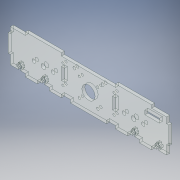
# Autodesk Inventor part: Soporte_Motor
Saved by Autodesk Inventor 2019 (Build 230136000, 136)
## iProperties
Created: 2020-04-02
Part Number: Soporte_Motor
Material: Generic
Document SubType Name: Modeling
Designer: Jurgen
Density: 1 g/cm^3
Appearance: Clear
Author: Jurgen
Autodesk Inventor part; units mm, degrees
ref_plane "YZ Plane" through (0, 0, 0) normal (1, 0, 0) x (0, 1, 0)
ref_plane "XZ Plane" through (0, 0, 0) normal (0, 1, 0) x (-1, 0, 0)
ref_plane "XY Plane" through (0, 0, 0) normal (0, 0, 1) x (1, 0, 0)
sketch "Sketch1" plane through (0, 0, 0) normal (0, 0, 1) x (1, 0, 0)
  arc A0 (19, -20) -> (20, -19) centre (19, -19) ccw construction
  line L0 (20, -19) -> (20, 19) construction
  arc A1 (20, 19) -> (19, 20) centre (19, 19) ccw construction
  line L1 (19, 20) -> (-19, 20) construction
  arc A2 (-19, 20) -> (-20, 19) centre (-19, 19) ccw construction
  line L2 (-20, 19) -> (-20, -19) construction
  arc A3 (-20, -19) -> (-19, -20) centre (-19, -19) ccw construction
  line L3 (-19, -20) -> (19, -20) construction
  circle A4 centre (-15.5, -15.5) radius 2
  circle A5 centre (15.5, -15.5) radius 2.2846
  circle A6 centre (15.5, 15.5) radius 2
  circle A7 centre (-15.5, 15.5) radius 2
  circle A8 centre (0, 0) radius 11
  line L4 (150, -20) -> (150, 20)
  line L5 (150, 20) -> (-150, 20)
  line L6 (-150, 20) -> (-150, -20)
  line L7 (-150, -20) -> (150, 20) construction
  line L8 (150, -20) -> (-150, 20) construction
  line L9 (50, -20) -> (100, -20) construction
  line L10 (100, -20) -> (100, -25)
  line L11 (100, -25) -> (50, -25)
  line L12 (50, -25) -> (50, -20)
  line L13 (100, -20) -> (150, -20)
  line L14 (-150, -20) -> (50, -20) construction
  line L15 (-150, -20) -> (-100, -20)
  line L16 (-100, -20) -> (-100, -25)
  line L17 (-100, -25) -> (-50, -25)
  line L18 (-50, -25) -> (-50, -20)
  line L19 (-50, -20) -> (50, -20)
  circle A9 centre (-91, 0) radius 3
  circle A10 centre (-59, 0) radius 3
  circle A11 centre (59, 0) radius 3
  circle A12 centre (91, 0) radius 3
  circle A13 centre (-75, 0) radius 4
  circle A14 centre (75, 0) radius 4
  dimension "d0" = 300
  dimension "d3" = 50
  dimension "d4" = 5
  dimension "d6" = 50
  dimension "d8" = 50
  dimension "d9" = 50
  dimension "d12" = 6
  dimension "d13" = 6
  dimension "d14" = 32
  dimension "d15" = 6
  dimension "d16" = 6
  dimension "d17" = 32
  dimension "d18" = 59
  dimension "d19" = 59
  dimension "d22" = 8
  dimension "d23" = 8
  dimension "d24" = 16
  dimension "d25" = 16
  constraints: 40 end point, 15 centre point, 8 point on circle, 5 perpendicular, 3 midpoint, 3 parallel, 2 horizontal, 2 point on line, 1 collinear
  measures "d0" distance of L5.end L4.end
  measures "d3" distance of L10.end L11.end
  measures "d4" distance of L9.end L10.end
  measures "d6" distance between parallel lines of L4 L10
  measures "d8" distance of L6.end L15.end
  measures "d9" distance of L16.end L17.end
  measures "d12" diameter of A9
  measures "d13" diameter of A10
  measures "d14" distance of A10.centre A9.centre
  measures "d15" diameter of A11
  measures "d16" diameter of A12
  measures "d17" distance of A12.centre A11.centre
  measures "d18" distance of point (0, 0) A10.centre
  measures "d19" distance of point (0, 0) A11.centre
  measures "d22" diameter of A13
  measures "d23" diameter of A14
  measures "d24" distance of A10.centre A13.centre
  measures "d25" distance of A14.centre A11.centre
extrude "Extrusion3" add sketch "Sketch1" along normal blind 5
sketch "Sketch2" plane through (0, 0, 5) normal (0, 0, 1) x (1, 0, 0)
  circle A0 centre (0, 0) radius 11 construction
  circle A1 centre (75, 0) radius 4 construction
  circle A2 centre (-75, 0) radius 4 construction
  circle A3 centre (91, 0) radius 3 construction
  circle A4 centre (59, 0) radius 3 construction
  circle A5 centre (-59, 0) radius 3 construction
  circle A6 centre (-91, 0) radius 3 construction
  circle A7 centre (15.5, -15.5) radius 2.2846 construction
  circle A8 centre (-15.5, 15.5) radius 2 construction
  circle A9 centre (15.5, 15.5) radius 2 construction
  circle A10 centre (-15.5, -15.5) radius 2 construction
  line L0 (-150, 20) -> (-150, -20) construction
  line L1 (-150, -20) -> (-100, -20) construction
  line L2 (-100, -20) -> (-100, -25) construction
  line L3 (-100, -25) -> (-50, -25) construction
  line L4 (-50, -25) -> (-50, -20) construction
  line L5 (-50, -20) -> (50, -20) construction
  line L6 (50, -20) -> (50, -25) construction
  line L7 (50, -25) -> (100, -25) construction
  line L8 (100, -25) -> (100, -20) construction
  line L9 (100, -20) -> (150, -20) construction
  line L10 (150, -20) -> (150, 20) construction
  line L11 (150, 20) -> (-150, 20) construction
  line L12 (150, 20) -> (-150, 20) construction
  line L13 (-150, 20) -> (150, 20)
  line L14 (150, 20) -> (150, 30)
  line L15 (-150, 30) -> (-150, 20)
  line L16 (-45, 30) -> (-45, 35)
  line L17 (-45, 35) -> (-105, 35) construction
  line L18 (-105, 35) -> (-105, 30)
  line L19 (45, 30) -> (45, 35)
  line L20 (45, 35) -> (105, 35) construction
  line L21 (105, 35) -> (105, 30)
  line L22 (-105, 30) -> (-150, 30)
  line L23 (150, 30) -> (105, 30)
  line L24 (45, 30) -> (-45, 30)
  line L25 (-105, 35) -> (-85, 35)
  line L26 (-65, 35) -> (-45, 35)
  line L27 (45, 35) -> (65, 35)
  line L28 (85, 35) -> (105, 35)
  line L29 (-85, 35) -> (-65, 35)
  line L30 (65, 35) -> (85, 35)
  point P0 (-120, 20)
  point P1 (70, 20)
  dimension "d42" = 10
  dimension "d43" = 5
  dimension "d44" = 5
  dimension "d57" = 45
  dimension "d58" = 90
  dimension "d59" = 45
  constraints: 36 end point, 6 parallel, 6 point on line, 2 collinear, 2 horizontal, 1 perpendicular
  measures "d42" distance of L14.end L13.end
  measures "d43" distance of L16.end L16.start
  measures "d44" distance of L19.start L19.end
  measures "d57" distance between parallel lines of L21 L14
  measures "d58" distance between parallel lines of L16 L19
  measures "d59" distance between parallel lines of L15 L18
extrude "Extrusion6" add sketch "Sketch2" against normal blind 5
sketch "Sketch4" plane through (0, 0, 5) normal (0, 0, 1) x (1, 0, 0)
  circle A0 centre (0, 0) radius 11 construction
  circle A1 centre (75, 0) radius 4 construction
  circle A2 centre (-75, 0) radius 4 construction
  circle A3 centre (91, 0) radius 3 construction
  circle A4 centre (59, 0) radius 3 construction
  circle A5 centre (-59, 0) radius 3 construction
  circle A6 centre (-91, 0) radius 3 construction
  circle A7 centre (15.5, -15.5) radius 2.2846 construction
  circle A8 centre (-15.5, 15.5) radius 2 construction
  circle A9 centre (15.5, 15.5) radius 2 construction
  circle A10 centre (-15.5, -15.5) radius 2 construction
  line L0 (-150, 30) -> (-150, -20) construction
  line L1 (-150, -20) -> (-100, -20) construction
  line L2 (-100, -20) -> (-100, -25) construction
  line L3 (-100, -25) -> (-50, -25) construction
  line L4 (-50, -25) -> (-50, -20) construction
  line L5 (-50, -20) -> (50, -20) construction
  line L6 (50, -20) -> (50, -25) construction
  line L7 (50, -25) -> (100, -25) construction
  line L8 (100, -25) -> (100, -20) construction
  line L9 (100, -20) -> (150, -20) construction
  line L10 (150, -20) -> (150, 30) construction
  line L11 (150, 30) -> (105, 30) construction
  line L12 (105, 30) -> (105, 35) construction
  line L13 (45, 35) -> (45, 30) construction
  line L14 (45, 30) -> (-45, 30) construction
  line L15 (-45, 30) -> (-45, 35) construction
  line L16 (-105, 35) -> (-105, 30) construction
  line L17 (-105, 30) -> (-150, 30) construction
  line L18 (-45, 0) -> (-45, 15) construction
  line L19 (-45, 15) -> (-40, 15) construction
  line L20 (-40, 15) -> (-40, -5) construction
  line L21 (-40, 15) -> (-45, 15)
  line L22 (-45, 15) -> (-45, -5)
  line L23 (-45, -5) -> (-40, -5)
  line L24 (-40, -5) -> (-40, 15)
  line L25 (45, 30) -> (-45, 30) construction
  line L26 (0, 30) -> (0, -20) construction
  line L27 (-50, -20) -> (50, -20) construction
  line L28 (45, 0) -> (45, 15) construction
  line L29 (45, 15) -> (40, 15) construction
  line L30 (40, 15) -> (40, -5) construction
  line L31 (40, 15) -> (45, 15)
  line L32 (45, 15) -> (45, -5)
  line L33 (45, -5) -> (40, -5)
  line L34 (40, -5) -> (40, 15)
  line L35 (105, 35) -> (45, 35) projected
  line L36 (-45, 35) -> (-105, 35) projected
  line L37 (0, 0) -> (-150, 0) construction
  line L38 (-150, 30) -> (-150, -20) construction
  line L39 (-42.5, 15) -> (-42.5, -5) construction
  line L40 (-42.5, 15) -> (-42.5, 30) construction
  line L41 (-45, 30) -> (45, 30) construction
  line L42 (-42.5, -5) -> (-42.5, -20) construction
  circle A11 centre (-42.5, -11) radius 2
  circle A12 centre (-42.5, 21) radius 2
  line L43 (45, 0) -> (45, 15) construction
  line L44 (45, 15) -> (40, 15) construction
  line L45 (40, 15) -> (40, -5) construction
  line L46 (40, 15) -> (45, 15)
  line L47 (45, 15) -> (45, -5)
  line L48 (45, -5) -> (40, -5)
  line L49 (40, -5) -> (40, 15)
  line L50 (42.5, 15) -> (42.5, -5) construction
  circle A13 centre (42.5, -11) radius 2
  circle A14 centre (42.5, 21) radius 2
  dimension "d48" = 5
  dimension "d50" = 40
  dimension "d98" = 20
  dimension "d103" = 15
  dimension "d104" = 6
  dimension "d105" = 6
  dimension "d106" = 4
  dimension "d107" = 4
  constraints: 54 end point, 15 symmetric about line, 7 point on line, 4 centre point, 4 midpoint, 4 perpendicular, 2 parallel, 1 horizontal, 1 vertical, 2 other
  measures "d48" distance of L18.end L19.end
  measures "d50" distance from line of point (0, 0) L20
  measures "d98" distance between parallel lines of L23 L19
  measures "d103" distance between parallel lines of L5 L23
  measures "d104" distance from line of A11.centre L23
  measures "d105" distance from line of L21 A12.centre
  measures "d106" diameter of A12
  measures "d107" diameter of A11
extrude "Extrusion7" cut sketch "Sketch4" against normal blind 5
sketch "Sketch7" plane through (100, -20, 0) normal (0, -1, 0) x (1, 0, 0)
  line L0 (50, 0) -> (0, 0) projected
  line L1 (50, 0) -> (50, 5) projected
  line L2 (0, 5) -> (50, 5) projected
  line L3 (0, 0) -> (0, 5) projected
  line L4 (-50, 0) -> (-150, 0) projected
  line L5 (-50, 0) -> (-50, 5) projected
  line L6 (-150, 5) -> (-50, 5) projected
  line L7 (-150, 0) -> (-150, 5) projected
  line L8 (-200, 0) -> (-250, 0) projected
  line L9 (-200, 0) -> (-250, 0) projected
  line L10 (-200, 0) -> (-200, 5) projected
  line L11 (-250, 5) -> (-200, 5) projected
  line L12 (-250, 0) -> (-250, 5) projected
  point P0 (-100, 0)
extrude "Extrusion9" add sketch "Sketch7" along normal blind 5
sketch "Sketch12" plane through (0, 0, 5) normal (0, 0, 1) x (1, 0, 0)
  line L0 (-45, -5) -> (-45, 15) construction
  line L1 (-45, 15) -> (-40, 15) construction
  line L2 (-40, 15) -> (-40, -5) construction
  line L3 (-40, -5) -> (-45, -5) construction
  line L4 (45, 15) -> (45, -5) construction
  line L5 (45, -5) -> (40, -5) construction
  line L6 (40, -5) -> (40, 15) construction
  line L7 (40, 15) -> (45, 15) construction
  circle A0 centre (0, 0) radius 11 construction
  circle A1 centre (75, 0) radius 4 construction
  circle A2 centre (-75, 0) radius 4 construction
  circle A3 centre (91, 0) radius 3 construction
  circle A4 centre (59, 0) radius 3 construction
  circle A5 centre (-59, 0) radius 3 construction
  circle A6 centre (-91, 0) radius 3 construction
  circle A7 centre (15.5, -15.5) radius 2.2846 construction
  circle A8 centre (-15.5, 15.5) radius 2 construction
  circle A9 centre (15.5, 15.5) radius 2 construction
  circle A10 centre (-15.5, -15.5) radius 2 construction
  line L8 (-150, 30) -> (-150, -25) construction
  line L9 (150, -25) -> (-150, -25) construction
  line L10 (150, 30) -> (150, -25) construction
  line L11 (150, 30) -> (105, 30) construction
  line L12 (105, 30) -> (105, 35) construction
  line L13 (105, 35) -> (45, 35) construction
  line L14 (45, 35) -> (45, 30) construction
  line L15 (45, 30) -> (-45, 30) construction
  line L16 (-45, 30) -> (-45, 35) construction
  line L17 (-45, 35) -> (-105, 35) construction
  line L18 (-105, 35) -> (-105, 30) construction
  line L19 (-105, 30) -> (-150, 30) construction
  line L20 (150, -25) -> (-150, -25) projected
  line L21 (-150, 30) -> (-130, 30)
  line L22 (-130, 30) -> (-130, -25)
  line L23 (-130, -25) -> (-150, -25)
  line L24 (-150, -25) -> (-150, 30)
  line L25 (105, 30) -> (150, 30) projected
  line L26 (150, 30) -> (130, 30)
  line L27 (130, 30) -> (130, -25)
  line L28 (130, -25) -> (150, -25)
  line L29 (150, -25) -> (150, 30)
  dimension "d79" = 20
  dimension "d80" = 20
  constraints: 16 end point, 4 parallel, 2 horizontal, 2 perpendicular, 2 point on line
  measures "d79" distance of L22.end L23.end
  measures "d80" distance of L28.end L27.end
extrude "Extrusion11" cut sketch "Sketch12" against normal blind 5
sketch "Sketch13" plane through (0, 0, 5) normal (0, 0, 1) x (1, 0, 0)
  line L0 (-130, 30) -> (-130, -25) construction
  line L1 (130, -25) -> (-130, -25) construction
  line L2 (130, -25) -> (130, 30) construction
  line L3 (130, 30) -> (105, 30) construction
  line L4 (105, 30) -> (105, 35) construction
  line L5 (105, 35) -> (45, 35) construction
  line L6 (45, 35) -> (45, 30) construction
  line L7 (45, 30) -> (-45, 30) construction
  line L8 (-45, 30) -> (-45, 35) construction
  line L9 (-45, 35) -> (-105, 35) construction
  line L10 (-105, 35) -> (-105, 30) construction
  line L11 (-105, 30) -> (-130, 30) construction
  line L12 (-45, -5) -> (-45, 15) construction
  line L13 (-45, 15) -> (-40, 15) construction
  line L14 (-40, 15) -> (-40, -5) construction
  line L15 (-40, -5) -> (-45, -5) construction
  line L16 (45, 15) -> (45, -5) construction
  line L17 (45, -5) -> (40, -5) construction
  line L18 (40, -5) -> (40, 15) construction
  line L19 (40, 15) -> (45, 15) construction
  circle A0 centre (0, 0) radius 11 construction
  circle A1 centre (75, 0) radius 4 construction
  circle A2 centre (-75, 0) radius 4 construction
  circle A3 centre (91, 0) radius 3 construction
  circle A4 centre (59, 0) radius 3 construction
  circle A5 centre (-59, 0) radius 3 construction
  circle A6 centre (-91, 0) radius 3 construction
  circle A7 centre (15.5, -15.5) radius 2.2846 construction
  circle A8 centre (-15.5, 15.5) radius 2 construction
  circle A9 centre (15.5, 15.5) radius 2 construction
  circle A10 centre (-15.5, -15.5) radius 2 construction
  line L20 (-105, 30) -> (-105, -25) construction
  line L21 (-45, 30) -> (-45, 35) construction
  line L22 (-45, 30) -> (-45, -25) construction
  line L23 (-45, 30) -> (45, 30) construction
  line L24 (45, 30) -> (45, -25) construction
  line L25 (105, 30) -> (105, -25) construction
  line L26 (-105, -25) -> (-45, -25) construction
  line L27 (-45, -25) -> (-45, -30) construction
  line L28 (-45, -30) -> (-105, -30) construction
  line L29 (-105, -30) -> (-105, -25) construction
  line L30 (45, -25) -> (105, -25) construction
  line L31 (105, -25) -> (105, -30) construction
  line L32 (105, -30) -> (45, -30) construction
  line L33 (45, -30) -> (45, -25) construction
  line L34 (-105, -25) -> (-85, -25)
  line L35 (-85, -25) -> (-85, -30)
  line L36 (-85, -30) -> (-105, -30)
  line L37 (-105, -30) -> (-105, -25)
  line L38 (-45, -25) -> (-65, -25)
  line L39 (-65, -25) -> (-65, -30)
  line L40 (-65, -30) -> (-45, -30)
  line L41 (-45, -30) -> (-45, -25)
  line L42 (45, -25) -> (65, -25)
  line L43 (65, -25) -> (65, -30)
  line L44 (65, -30) -> (45, -30)
  line L45 (45, -30) -> (45, -25)
  line L46 (105, -25) -> (85, -25)
  line L47 (85, -25) -> (85, -30)
  line L48 (85, -30) -> (105, -30)
  line L49 (105, -30) -> (105, -25)
  dimension "d83" = 5
  dimension "d84" = 5
  dimension "d85" = 20
  dimension "d86" = 20
  dimension "d87" = 20
  dimension "d88" = 20
  constraints: 56 end point, 12 parallel, 10 perpendicular, 8 point on line, 6 horizontal
  measures "d83" distance of L26.end L27.end
  measures "d84" distance of L30.end L31.end
  measures "d85" distance of L35.end L36.end
  measures "d86" distance of L40.end L39.end
  measures "d87" distance of L43.end L44.end
  measures "d88" distance of L48.end L47.end
extrude "Extrusion12" add sketch "Sketch13" against normal blind 5
sketch "Sketch14" plane through (0, 0, 5) normal (0, 0, 1) x (1, 0, 0)
  line L0 (-130, 30) -> (-130, -25) construction
  line L1 (-105, -25) -> (-130, -25) construction
  line L2 (-105, -30) -> (-105, -25) construction
  line L3 (-85, -30) -> (-105, -30) construction
  line L4 (-85, -25) -> (-85, -30) construction
  line L5 (-65, -25) -> (-85, -25) construction
  line L6 (-65, -25) -> (-65, -30) construction
  line L7 (-65, -30) -> (-45, -30) construction
  line L8 (-45, -30) -> (-45, -25) construction
  line L9 (45, -25) -> (-45, -25) construction
  line L10 (45, -30) -> (45, -25) construction
  line L11 (65, -30) -> (45, -30) construction
  line L12 (65, -25) -> (65, -30) construction
  line L13 (85, -25) -> (65, -25) construction
  line L14 (85, -25) -> (85, -30) construction
  line L15 (85, -30) -> (105, -30) construction
  line L16 (105, -30) -> (105, -25) construction
  line L17 (130, -25) -> (105, -25) construction
  line L18 (130, -25) -> (130, 30) construction
  line L19 (130, 30) -> (105, 30) construction
  line L20 (105, 30) -> (105, 35) construction
  line L21 (105, 35) -> (45, 35) construction
  line L22 (45, 35) -> (45, 30) construction
  line L23 (45, 30) -> (-45, 30) construction
  line L24 (-45, 30) -> (-45, 35) construction
  line L25 (-45, 35) -> (-105, 35) construction
  line L26 (-105, 35) -> (-105, 30) construction
  line L27 (-105, 30) -> (-130, 30) construction
  line L28 (-45, -5) -> (-45, 15) construction
  line L29 (-45, 15) -> (-40, 15) construction
  line L30 (-40, 15) -> (-40, -5) construction
  line L31 (-40, -5) -> (-45, -5) construction
  line L32 (45, 15) -> (45, -5) construction
  line L33 (45, -5) -> (40, -5) construction
  line L34 (40, -5) -> (40, 15) construction
  line L35 (40, 15) -> (45, 15) construction
  circle A0 centre (0, 0) radius 11 construction
  circle A1 centre (75, 0) radius 4 construction
  circle A2 centre (-75, 0) radius 4 construction
  circle A3 centre (91, 0) radius 3 construction
  circle A4 centre (59, 0) radius 3 construction
  circle A5 centre (-59, 0) radius 3 construction
  circle A6 centre (-91, 0) radius 3 construction
  circle A7 centre (15.5, -15.5) radius 2.2846 construction
  circle A8 centre (-15.5, 15.5) radius 2 construction
  circle A9 centre (15.5, 15.5) radius 2 construction
  circle A10 centre (-15.5, -15.5) radius 2 construction
  line L36 (-85, -25) -> (-77, -25) construction
  line L37 (-65, -25) -> (-85, -25) construction
  line L38 (-77, -25) -> (-73, -25) construction
  line L39 (-73, -25) -> (-73, -15) construction
  line L40 (-73, -15) -> (-77, -15) construction
  line L41 (-77, -15) -> (-77, -25) construction
  line L42 (-75, -15) -> (-75, -25) construction
  line L43 (-71, -22) -> (-79, -22) construction
  line L44 (-79, -22) -> (-79, -18) construction
  line L45 (-79, -18) -> (-71, -18) construction
  line L46 (-71, -18) -> (-71, -22) construction
  line L47 (-71, -22) -> (-79, -18) construction
  line L48 (-79, -22) -> (-71, -18) construction
  line L49 (-73, -25) -> (-77, -25)
  line L50 (-77, -25) -> (-77, -22)
  line L51 (-77, -22) -> (-79, -22)
  line L52 (-79, -22) -> (-79, -18)
  line L53 (-79, -18) -> (-77, -18)
  line L54 (-77, -18) -> (-77, -15)
  line L55 (-77, -15) -> (-73, -15)
  line L56 (-73, -15) -> (-73, -18)
  line L57 (-73, -18) -> (-71, -18)
  line L58 (-71, -18) -> (-71, -22)
  line L59 (-71, -22) -> (-73, -22)
  line L60 (-73, -22) -> (-73, -25)
  line L61 (-85, -30) -> (-105, -30) construction
  line L62 (-95, -30) -> (-95, 35) construction
  line L63 (-45, 30) -> (45, 30) construction
  line L64 (0, 30) -> (0, -25) construction
  line L65 (-113, -25) -> (-117, -25) construction
  line L66 (-117, -25) -> (-117, -15) construction
  line L67 (-117, -15) -> (-113, -15) construction
  line L68 (-113, -15) -> (-113, -25) construction
  line L69 (-115, -15) -> (-115, -25) construction
  line L70 (-119, -22) -> (-111, -22) construction
  line L71 (-111, -22) -> (-111, -18) construction
  line L72 (-111, -18) -> (-119, -18) construction
  line L73 (-119, -18) -> (-119, -22) construction
  line L74 (-119, -22) -> (-111, -18) construction
  line L75 (-111, -22) -> (-119, -18) construction
  line L76 (-117, -25) -> (-113, -25)
  line L77 (-113, -25) -> (-113, -22)
  line L78 (-113, -22) -> (-111, -22)
  line L79 (-111, -22) -> (-111, -18)
  line L80 (-111, -18) -> (-113, -18)
  line L81 (-113, -18) -> (-113, -15)
  line L82 (-113, -15) -> (-117, -15)
  line L83 (-117, -15) -> (-117, -18)
  line L84 (-117, -18) -> (-119, -18)
  line L85 (-119, -18) -> (-119, -22)
  line L86 (-119, -22) -> (-117, -22)
  line L87 (-117, -22) -> (-117, -25)
  line L88 (85, -25) -> (77, -25) construction
  line L89 (77, -25) -> (73, -25) construction
  line L90 (73, -25) -> (73, -15) construction
  line L91 (73, -15) -> (77, -15) construction
  line L92 (77, -15) -> (77, -25) construction
  line L93 (75, -15) -> (75, -25) construction
  line L94 (71, -22) -> (79, -22) construction
  line L95 (79, -22) -> (79, -18) construction
  line L96 (79, -18) -> (71, -18) construction
  line L97 (71, -18) -> (71, -22) construction
  line L98 (71, -22) -> (79, -18) construction
  line L99 (79, -22) -> (71, -18) construction
  line L100 (73, -25) -> (77, -25)
  line L101 (77, -25) -> (77, -22)
  line L102 (77, -22) -> (79, -22)
  line L103 (79, -22) -> (79, -18)
  line L104 (79, -18) -> (77, -18)
  line L105 (77, -18) -> (77, -15)
  line L106 (77, -15) -> (73, -15)
  line L107 (73, -15) -> (73, -18)
  line L108 (73, -18) -> (71, -18)
  line L109 (71, -18) -> (71, -22)
  line L110 (71, -22) -> (73, -22)
  line L111 (73, -22) -> (73, -25)
  line L112 (119, -22) -> (117, -22)
  line L113 (113, -22) -> (111, -22)
  line L114 (119, -22) -> (111, -22) construction
  line L115 (111, -18) -> (113, -18)
  line L116 (111, -18) -> (119, -18) construction
  line L117 (111, -22) -> (111, -18) construction
  line L118 (111, -22) -> (111, -18)
  line L119 (111, -22) -> (119, -18) construction
  line L120 (119, -22) -> (111, -18) construction
  line L121 (117, -25) -> (117, -15) construction
  line L122 (113, -15) -> (113, -25) construction
  line L123 (115, -15) -> (115, -25) construction
  line L124 (117, -18) -> (119, -18)
  line L125 (119, -18) -> (119, -22)
  line L126 (117, -15) -> (113, -15) construction
  line L127 (113, -18) -> (113, -15)
  line L128 (117, -15) -> (117, -18)
  line L129 (119, -18) -> (119, -22) construction
  line L130 (113, -25) -> (117, -25) construction
  line L131 (113, -25) -> (113, -22)
  line L132 (117, -25) -> (113, -25)
  line L133 (117, -22) -> (117, -25)
  line L134 (113, -15) -> (117, -15)
  point P0 (-75, -20)
  point P1 (-115, -20)
  point P2 (75, -20)
  point P3 (115, -20)
  dimension "d91" = 8
  dimension "d92" = 4
  dimension "d93" = 10
  dimension "d94" = 8
  dimension "d95" = 4
  constraints: 192 end point, 45 symmetric about line, 34 point on line, 14 midpoint, 7 perpendicular, 4 parallel, 3 collinear, 3 horizontal
  measures "d91" distance of L4.start L36.end
  measures "d92" distance of L40.end L39.end
  measures "d93" distance of L39.end L38.end
  measures "d94" distance of L44.end L45.end
  measures "d95" distance of L43.end L44.end
extrude "Extrusion13" cut sketch "Sketch14" against normal blind 5
sketch "Sketch15" plane through (0, 0, 5) normal (0, 0, 1) x (1, 0, 0)
  line L0 (77, -22) -> (77, -25) construction
  line L1 (85, -25) -> (77, -25) construction
  line L2 (85, -25) -> (85, -30) construction
  line L3 (85, -30) -> (105, -30) construction
  line L4 (105, -30) -> (105, -25) construction
  line L5 (113, -25) -> (105, -25) construction
  line L6 (113, -25) -> (113, -22) construction
  line L7 (113, -22) -> (111, -22) construction
  line L8 (111, -22) -> (111, -18) construction
  line L9 (111, -18) -> (113, -18) construction
  line L10 (113, -18) -> (113, -15) construction
  line L11 (113, -15) -> (117, -15) construction
  line L12 (117, -15) -> (117, -18) construction
  line L13 (117, -18) -> (119, -18) construction
  line L14 (119, -18) -> (119, -22) construction
  line L15 (119, -22) -> (117, -22) construction
  line L16 (117, -22) -> (117, -25) construction
  line L17 (130, -25) -> (117, -25) construction
  line L18 (130, -25) -> (130, 30) construction
  line L19 (130, 30) -> (105, 30) construction
  line L20 (105, 30) -> (105, 35) construction
  line L21 (105, 35) -> (45, 35) construction
  line L22 (45, 35) -> (45, 30) construction
  line L23 (45, 30) -> (-45, 30) construction
  line L24 (-45, 30) -> (-45, 35) construction
  line L25 (-45, 35) -> (-105, 35) construction
  line L26 (-105, 35) -> (-105, 30) construction
  line L27 (-105, 30) -> (-130, 30) construction
  line L28 (-130, 30) -> (-130, -25) construction
  line L29 (-117, -25) -> (-130, -25) construction
  line L30 (-117, -25) -> (-117, -22) construction
  line L31 (-117, -22) -> (-119, -22) construction
  line L32 (-119, -22) -> (-119, -18) construction
  line L33 (-119, -18) -> (-117, -18) construction
  line L34 (-117, -18) -> (-117, -15) construction
  line L35 (-117, -15) -> (-113, -15) construction
  line L36 (-113, -15) -> (-113, -18) construction
  line L37 (-113, -18) -> (-111, -18) construction
  line L38 (-111, -18) -> (-111, -22) construction
  line L39 (-111, -22) -> (-113, -22) construction
  line L40 (-113, -22) -> (-113, -25) construction
  line L41 (-105, -25) -> (-113, -25) construction
  line L42 (-105, -30) -> (-105, -25) construction
  line L43 (-85, -30) -> (-105, -30) construction
  line L44 (-85, -25) -> (-85, -30) construction
  line L45 (-77, -25) -> (-85, -25) construction
  line L46 (-77, -25) -> (-77, -22) construction
  line L47 (-77, -22) -> (-79, -22) construction
  line L48 (-79, -22) -> (-79, -18) construction
  line L49 (-79, -18) -> (-77, -18) construction
  line L50 (-77, -18) -> (-77, -15) construction
  line L51 (-77, -15) -> (-73, -15) construction
  line L52 (-73, -15) -> (-73, -18) construction
  line L53 (-73, -18) -> (-71, -18) construction
  line L54 (-71, -18) -> (-71, -22) construction
  line L55 (-71, -22) -> (-73, -22) construction
  line L56 (-73, -22) -> (-73, -25) construction
  line L57 (-65, -25) -> (-73, -25) construction
  line L58 (-65, -25) -> (-65, -30) construction
  line L59 (-65, -30) -> (-45, -30) construction
  line L60 (-45, -30) -> (-45, -25) construction
  line L61 (45, -25) -> (-45, -25) construction
  line L62 (45, -30) -> (45, -25) construction
  line L63 (65, -30) -> (45, -30) construction
  line L64 (65, -25) -> (65, -30) construction
  line L65 (73, -25) -> (65, -25) construction
  line L66 (73, -25) -> (73, -22) construction
  line L67 (73, -22) -> (71, -22) construction
  line L68 (71, -22) -> (71, -18) construction
  line L69 (71, -18) -> (73, -18) construction
  line L70 (73, -18) -> (73, -15) construction
  line L71 (73, -15) -> (77, -15) construction
  line L72 (77, -15) -> (77, -18) construction
  line L73 (77, -18) -> (79, -18) construction
  line L74 (79, -18) -> (79, -22) construction
  line L75 (79, -22) -> (77, -22) construction
  line L76 (-45, -5) -> (-45, 15) construction
  line L77 (-45, 15) -> (-40, 15) construction
  line L78 (-40, 15) -> (-40, -5) construction
  line L79 (-40, -5) -> (-45, -5) construction
  circle A0 centre (42.5, 21) radius 2 construction
  circle A1 centre (-42.5, -11) radius 2 construction
  circle A2 centre (-42.5, 21) radius 2 construction
  circle A3 centre (42.5, -11) radius 2 construction
  line L80 (45, 15) -> (45, -5) construction
  line L81 (45, -5) -> (40, -5) construction
  line L82 (40, -5) -> (40, 15) construction
  line L83 (40, 15) -> (45, 15) construction
  circle A4 centre (0, 0) radius 11 construction
  circle A5 centre (75, 0) radius 4 construction
  circle A6 centre (-75, 0) radius 4 construction
  circle A7 centre (91, 0) radius 3 construction
  circle A8 centre (59, 0) radius 3 construction
  circle A9 centre (-59, 0) radius 3 construction
  circle A10 centre (-91, 0) radius 3 construction
  circle A11 centre (15.5, -15.5) radius 2.2846 construction
  circle A12 centre (-15.5, 15.5) radius 2 construction
  circle A13 centre (15.5, 15.5) radius 2 construction
  circle A14 centre (-15.5, -15.5) radius 2 construction
  line L84 (23.5, -23.5) -> (-23.5, -23.5) construction
  line L85 (-23.5, -23.5) -> (-23.5, 23.5) construction
  line L86 (-23.5, 23.5) -> (23.5, 23.5) construction
  line L87 (23.5, 23.5) -> (23.5, -23.5) construction
  line L88 (23.5, -23.5) -> (-23.5, 23.5) construction
  line L89 (-23.5, -23.5) -> (23.5, 23.5) construction
  circle A15 centre (-23.5, 23.5) radius 2.5 construction
  circle A16 centre (23.5, 23.5) radius 2.5 construction
  circle A17 centre (-23.5, -23.5) radius 2.5 construction
  circle A18 centre (23.5, -23.5) radius 2.5 construction
  line L90 (-30, -25) -> (30, -25)
  line L91 (30, -25) -> (30, -30)
  line L92 (30, -30) -> (-30, -30)
  line L93 (-30, -30) -> (-30, -25)
  dimension "d108" = 47
  dimension "d109" = 47
  dimension "d110" = 5
  dimension "d111" = 5
  dimension "d112" = 5
  dimension "d113" = 5
  dimension "d114" = 60
  dimension "d115" = 5
  dimension "d116" = 15
  constraints: 20 end point, 4 centre point, 4 coincident, 4 parallel, 2 horizontal, 2 midpoint, 2 perpendicular, 1 point on line
  measures "d108" distance of L85.end L86.end
  measures "d109" distance of L84.end L85.end
  measures "d110" diameter of A15
  measures "d111" diameter of A16
  measures "d112" diameter of A17
  measures "d113" diameter of A18
  measures "d114" distance of L91.end L92.end
  measures "d115" distance of L90.end L91.end
  measures "d116" distance between parallel lines of L93 L60
extrude "Extrusion14" add sketch "Sketch15" against normal blind 5
sketch "Sketch16" plane through (0, 0, 5) normal (0, 0, 1) x (1, 0, 0)
  line L0 (77, -22) -> (77, -25) construction
  line L1 (85, -25) -> (77, -25) construction
  line L2 (85, -25) -> (85, -30) construction
  line L3 (85, -30) -> (105, -30) construction
  line L4 (105, -30) -> (105, -25) construction
  line L5 (113, -25) -> (105, -25) construction
  line L6 (113, -25) -> (113, -22) construction
  line L7 (113, -22) -> (111, -22) construction
  line L8 (111, -22) -> (111, -18) construction
  line L9 (111, -18) -> (113, -18) construction
  line L10 (113, -18) -> (113, -15) construction
  line L11 (113, -15) -> (117, -15) construction
  line L12 (117, -15) -> (117, -18) construction
  line L13 (117, -18) -> (119, -18) construction
  line L14 (119, -18) -> (119, -22) construction
  line L15 (119, -22) -> (117, -22) construction
  line L16 (117, -22) -> (117, -25) construction
  line L17 (130, -25) -> (117, -25) construction
  line L18 (130, -25) -> (130, 30) construction
  line L19 (130, 30) -> (105, 30) construction
  line L20 (105, 30) -> (105, 35) construction
  line L21 (105, 35) -> (45, 35) construction
  line L22 (45, 35) -> (45, 30) construction
  line L23 (45, 30) -> (-45, 30) construction
  line L24 (-45, 30) -> (-45, 35) construction
  line L25 (-45, 35) -> (-105, 35) construction
  line L26 (-105, 35) -> (-105, 30) construction
  line L27 (-105, 30) -> (-130, 30) construction
  line L28 (-130, 30) -> (-130, -25) construction
  line L29 (-117, -25) -> (-130, -25) construction
  line L30 (-117, -25) -> (-117, -22) construction
  line L31 (-117, -22) -> (-119, -22) construction
  line L32 (-119, -22) -> (-119, -18) construction
  line L33 (-119, -18) -> (-117, -18) construction
  line L34 (-117, -18) -> (-117, -15) construction
  line L35 (-117, -15) -> (-113, -15) construction
  line L36 (-113, -15) -> (-113, -18) construction
  line L37 (-113, -18) -> (-111, -18) construction
  line L38 (-111, -18) -> (-111, -22) construction
  line L39 (-111, -22) -> (-113, -22) construction
  line L40 (-113, -22) -> (-113, -25) construction
  line L41 (-105, -25) -> (-113, -25) construction
  line L42 (-105, -30) -> (-105, -25) construction
  line L43 (-85, -30) -> (-105, -30) construction
  line L44 (-85, -25) -> (-85, -30) construction
  line L45 (-77, -25) -> (-85, -25) construction
  line L46 (-77, -25) -> (-77, -22) construction
  line L47 (-77, -22) -> (-79, -22) construction
  line L48 (-79, -22) -> (-79, -18) construction
  line L49 (-79, -18) -> (-77, -18) construction
  line L50 (-77, -18) -> (-77, -15) construction
  line L51 (-77, -15) -> (-73, -15) construction
  line L52 (-73, -15) -> (-73, -18) construction
  line L53 (-73, -18) -> (-71, -18) construction
  line L54 (-71, -18) -> (-71, -22) construction
  line L55 (-71, -22) -> (-73, -22) construction
  line L56 (-73, -22) -> (-73, -25) construction
  line L57 (-65, -25) -> (-73, -25) construction
  line L58 (-65, -25) -> (-65, -30) construction
  line L59 (-65, -30) -> (-45, -30) construction
  line L60 (-45, -30) -> (-45, -25) construction
  line L61 (45, -25) -> (-45, -25) construction
  line L62 (45, -30) -> (45, -25) construction
  line L63 (65, -30) -> (45, -30) construction
  line L64 (65, -25) -> (65, -30) construction
  line L65 (73, -25) -> (65, -25) construction
  line L66 (73, -25) -> (73, -22) construction
  line L67 (73, -22) -> (71, -22) construction
  line L68 (71, -22) -> (71, -18) construction
  line L69 (71, -18) -> (73, -18) construction
  line L70 (73, -18) -> (73, -15) construction
  line L71 (73, -15) -> (77, -15) construction
  line L72 (77, -15) -> (77, -18) construction
  line L73 (77, -18) -> (79, -18) construction
  line L74 (79, -18) -> (79, -22) construction
  line L75 (79, -22) -> (77, -22) construction
  line L76 (-45, -5) -> (-45, 15) construction
  line L77 (-45, 15) -> (-40, 15) construction
  line L78 (-40, 15) -> (-40, -5) construction
  line L79 (-40, -5) -> (-45, -5) construction
  circle A0 centre (42.5, 21) radius 2 construction
  circle A1 centre (-42.5, -11) radius 2 construction
  circle A2 centre (-42.5, 21) radius 2 construction
  circle A3 centre (42.5, -11) radius 2 construction
  line L80 (45, 15) -> (45, -5) construction
  line L81 (45, -5) -> (40, -5) construction
  line L82 (40, -5) -> (40, 15) construction
  line L83 (40, 15) -> (45, 15) construction
  circle A4 centre (0, 0) radius 11 construction
  circle A5 centre (75, 0) radius 4 construction
  circle A6 centre (-75, 0) radius 4 construction
  circle A7 centre (91, 0) radius 3 construction
  circle A8 centre (59, 0) radius 3 construction
  circle A9 centre (-59, 0) radius 3 construction
  circle A10 centre (-91, 0) radius 3 construction
  circle A11 centre (15.5, -15.5) radius 2.2846 construction
  circle A12 centre (-15.5, 15.5) radius 2 construction
  circle A13 centre (15.5, 15.5) radius 2 construction
  circle A14 centre (-15.5, -15.5) radius 2 construction
  line L84 (23.5, -23.5) -> (-23.5, -23.5) construction
  line L85 (-23.5, -23.5) -> (-23.5, 23.5) construction
  line L86 (-23.5, 23.5) -> (23.5, 23.5) construction
  line L87 (23.5, 23.5) -> (23.5, -23.5) construction
  line L88 (23.5, -23.5) -> (-23.5, 23.5) construction
  line L89 (-23.5, -23.5) -> (23.5, 23.5) construction
  circle A15 centre (-23.5, 23.5) radius 2.5
  circle A16 centre (23.5, 23.5) radius 2.5
  line L90 (-30, -25) -> (30, -25) construction
  line L91 (30, -25) -> (30, -30) construction
  line L92 (30, -30) -> (-30, -30) construction
  line L93 (-30, -30) -> (-30, -25) construction
  dimension "d119" = 47
  dimension "d120" = 47
  dimension "d121" = 5
  dimension "d122" = 5
  dimension "d125" = 60
  dimension "d126" = 5
  dimension "d127" = 15
  constraints: 188 end point, 17 centre point, 4 parallel, 2 coincident, 2 horizontal, 2 midpoint, 2 perpendicular, 1 point on line
  measures "d119" distance of L85.end L86.end
  measures "d120" distance of L84.end L85.end
  measures "d121" diameter of A15
  measures "d122" diameter of A16
  measures "d125" distance of L91.end L92.end
  measures "d126" distance of L90.end L91.end
  measures "d127" distance between parallel lines of L93 L60
extrude "Extrusion16" cut sketch "Sketch16" against normal blind 5
sketch "Sketch17" plane through (0, 0, 5) normal (0, 0, 1) x (1, 0, 0)
  circle A0 centre (-23.5, 23.5) radius 2.5 construction
  circle A1 centre (23.5, 23.5) radius 2.5 construction
  line L0 (77, -22) -> (77, -25) construction
  line L1 (85, -25) -> (77, -25) construction
  line L2 (85, -25) -> (85, -30) construction
  line L3 (85, -30) -> (105, -30) construction
  line L4 (105, -30) -> (105, -25) construction
  line L5 (113, -25) -> (105, -25) construction
  line L6 (113, -25) -> (113, -22) construction
  line L7 (113, -22) -> (111, -22) construction
  line L8 (111, -22) -> (111, -18) construction
  line L9 (111, -18) -> (113, -18) construction
  line L10 (113, -18) -> (113, -15) construction
  line L11 (113, -15) -> (117, -15) construction
  line L12 (117, -15) -> (117, -18) construction
  line L13 (117, -18) -> (119, -18) construction
  line L14 (119, -18) -> (119, -22) construction
  line L15 (119, -22) -> (117, -22) construction
  line L16 (117, -22) -> (117, -25) construction
  line L17 (130, -25) -> (117, -25) construction
  line L18 (130, -25) -> (130, 30) construction
  line L19 (130, 30) -> (105, 30) construction
  line L20 (105, 30) -> (105, 35) construction
  line L21 (105, 35) -> (45, 35) construction
  line L22 (45, 35) -> (45, 30) construction
  line L23 (45, 30) -> (-45, 30) construction
  line L24 (-45, 30) -> (-45, 35) construction
  line L25 (-45, 35) -> (-105, 35) construction
  line L26 (-105, 35) -> (-105, 30) construction
  line L27 (-105, 30) -> (-130, 30) construction
  line L28 (-130, 30) -> (-130, -25) construction
  line L29 (-117, -25) -> (-130, -25) construction
  line L30 (-117, -25) -> (-117, -22) construction
  line L31 (-117, -22) -> (-119, -22) construction
  line L32 (-119, -22) -> (-119, -18) construction
  line L33 (-119, -18) -> (-117, -18) construction
  line L34 (-117, -18) -> (-117, -15) construction
  line L35 (-117, -15) -> (-113, -15) construction
  line L36 (-113, -15) -> (-113, -18) construction
  line L37 (-113, -18) -> (-111, -18) construction
  line L38 (-111, -18) -> (-111, -22) construction
  line L39 (-111, -22) -> (-113, -22) construction
  line L40 (-113, -22) -> (-113, -25) construction
  line L41 (-105, -25) -> (-113, -25) construction
  line L42 (-105, -30) -> (-105, -25) construction
  line L43 (-85, -30) -> (-105, -30) construction
  line L44 (-85, -25) -> (-85, -30) construction
  line L45 (-77, -25) -> (-85, -25) construction
  line L46 (-77, -25) -> (-77, -22) construction
  line L47 (-77, -22) -> (-79, -22) construction
  line L48 (-79, -22) -> (-79, -18) construction
  line L49 (-79, -18) -> (-77, -18) construction
  line L50 (-77, -18) -> (-77, -15) construction
  line L51 (-77, -15) -> (-73, -15) construction
  line L52 (-73, -15) -> (-73, -18) construction
  line L53 (-73, -18) -> (-71, -18) construction
  line L54 (-71, -18) -> (-71, -22) construction
  line L55 (-71, -22) -> (-73, -22) construction
  line L56 (-73, -22) -> (-73, -25) construction
  line L57 (-65, -25) -> (-73, -25) construction
  line L58 (-65, -25) -> (-65, -30) construction
  line L59 (-65, -30) -> (-45, -30) construction
  line L60 (-45, -30) -> (-45, -25) construction
  line L61 (-30, -25) -> (-45, -25) construction
  line L62 (-30, -30) -> (-30, -25) construction
  line L63 (30, -30) -> (-30, -30) construction
  line L64 (30, -25) -> (30, -30) construction
  line L65 (45, -25) -> (30, -25) construction
  line L66 (45, -30) -> (45, -25) construction
  line L67 (65, -30) -> (45, -30) construction
  line L68 (65, -25) -> (65, -30) construction
  line L69 (73, -25) -> (65, -25) construction
  line L70 (73, -25) -> (73, -22) construction
  line L71 (73, -22) -> (71, -22) construction
  line L72 (71, -22) -> (71, -18) construction
  line L73 (71, -18) -> (73, -18) construction
  line L74 (73, -18) -> (73, -15) construction
  line L75 (73, -15) -> (77, -15) construction
  line L76 (77, -15) -> (77, -18) construction
  line L77 (77, -18) -> (79, -18) construction
  line L78 (79, -18) -> (79, -22) construction
  line L79 (79, -22) -> (77, -22) construction
  line L80 (-45, -5) -> (-45, 15) construction
  line L81 (-45, 15) -> (-40, 15) construction
  line L82 (-40, 15) -> (-40, -5) construction
  line L83 (-40, -5) -> (-45, -5) construction
  circle A2 centre (42.5, 21) radius 2 construction
  circle A3 centre (-42.5, -11) radius 2 construction
  circle A4 centre (-42.5, 21) radius 2 construction
  circle A5 centre (42.5, -11) radius 2 construction
  line L84 (45, 15) -> (45, -5) construction
  line L85 (45, -5) -> (40, -5) construction
  line L86 (40, -5) -> (40, 15) construction
  line L87 (40, 15) -> (45, 15) construction
  circle A6 centre (0, 0) radius 11 construction
  circle A7 centre (75, 0) radius 4 construction
  circle A8 centre (-75, 0) radius 4 construction
  circle A9 centre (91, 0) radius 3 construction
  circle A10 centre (59, 0) radius 3 construction
  circle A11 centre (-59, 0) radius 3 construction
  circle A12 centre (-91, 0) radius 3 construction
  circle A13 centre (15.5, -15.5) radius 2.2846 construction
  circle A14 centre (-15.5, 15.5) radius 2 construction
  circle A15 centre (15.5, 15.5) radius 2 construction
  circle A16 centre (-15.5, -15.5) radius 2 construction
  line L88 (-130, 30) -> (-130, -25) construction
  line L89 (-130, 20) -> (-133.5, 20)
  line L90 (-133.5, 20) -> (-133.5, -10)
  line L91 (-133.5, -10) -> (-130, -10)
  line L92 (-130, -10) -> (-130, 20)
  line L93 (0, 30) -> (0, -30) construction
  line L94 (130, 20) -> (133.5, 20)
  line L95 (133.5, 20) -> (133.5, -10)
  line L96 (133.5, -10) -> (130, -10)
  line L97 (130, -10) -> (130, 20)
  dimension "d132" = 3.5
  dimension "d133" = 30
  dimension "d134" = 10
  constraints: 18 end point, 4 symmetric about line, 2 midpoint, 2 parallel, 1 horizontal, 1 perpendicular, 1 point on line
  measures "d132" distance of L91.end L90.end
  measures "d133" distance of L90.end L89.end
  measures "d134" distance between parallel lines of L27 L89
extrude "Extrusion17" add sketch "Sketch17" against normal blind 5
sketch "Sketch18" plane through (0, 0, 5) normal (0, 0, 1) x (1, 0, 0)
  circle A0 centre (-23.5, 23.5) radius 2.5 construction
  circle A1 centre (23.5, 23.5) radius 2.5 construction
  line L0 (77, -22) -> (77, -25) construction
  line L1 (85, -25) -> (77, -25) construction
  line L2 (85, -25) -> (85, -30) construction
  line L3 (85, -30) -> (105, -30) construction
  line L4 (105, -30) -> (105, -25) construction
  line L5 (113, -25) -> (105, -25) construction
  line L6 (113, -25) -> (113, -22) construction
  line L7 (113, -22) -> (111, -22) construction
  line L8 (111, -22) -> (111, -18) construction
  line L9 (111, -18) -> (113, -18) construction
  line L10 (113, -18) -> (113, -15) construction
  line L11 (113, -15) -> (117, -15) construction
  line L12 (117, -15) -> (117, -18) construction
  line L13 (117, -18) -> (119, -18) construction
  line L14 (119, -18) -> (119, -22) construction
  line L15 (119, -22) -> (117, -22) construction
  line L16 (117, -22) -> (117, -25) construction
  line L17 (130, -25) -> (117, -25) construction
  line L18 (130, -25) -> (130, -10) construction
  line L19 (130, -10) -> (133.5, -10) construction
  line L20 (133.5, -10) -> (133.5, 20) construction
  line L21 (133.5, 20) -> (130, 20) construction
  line L22 (130, 20) -> (130, 30) construction
  line L23 (130, 30) -> (105, 30) construction
  line L24 (105, 30) -> (105, 35) construction
  line L25 (105, 35) -> (45, 35) construction
  line L26 (45, 35) -> (45, 30) construction
  line L27 (45, 30) -> (-45, 30) construction
  line L28 (-45, 30) -> (-45, 35) construction
  line L29 (-45, 35) -> (-105, 35) construction
  line L30 (-105, 35) -> (-105, 30) construction
  line L31 (-105, 30) -> (-130, 30) construction
  line L32 (-130, 30) -> (-130, 20) construction
  line L33 (-130, 20) -> (-133.5, 20) construction
  line L34 (-133.5, 20) -> (-133.5, -10) construction
  line L35 (-133.5, -10) -> (-130, -10) construction
  line L36 (-130, -10) -> (-130, -25) construction
  line L37 (-117, -25) -> (-130, -25) construction
  line L38 (-117, -25) -> (-117, -22) construction
  line L39 (-117, -22) -> (-119, -22) construction
  line L40 (-119, -22) -> (-119, -18) construction
  line L41 (-119, -18) -> (-117, -18) construction
  line L42 (-117, -18) -> (-117, -15) construction
  line L43 (-117, -15) -> (-113, -15) construction
  line L44 (-113, -15) -> (-113, -18) construction
  line L45 (-113, -18) -> (-111, -18) construction
  line L46 (-111, -18) -> (-111, -22) construction
  line L47 (-111, -22) -> (-113, -22) construction
  line L48 (-113, -22) -> (-113, -25) construction
  line L49 (-105, -25) -> (-113, -25) construction
  line L50 (-105, -30) -> (-105, -25) construction
  line L51 (-85, -30) -> (-105, -30) construction
  line L52 (-85, -25) -> (-85, -30) construction
  line L53 (-77, -25) -> (-85, -25) construction
  line L54 (-77, -25) -> (-77, -22) construction
  line L55 (-77, -22) -> (-79, -22) construction
  line L56 (-79, -22) -> (-79, -18) construction
  line L57 (-79, -18) -> (-77, -18) construction
  line L58 (-77, -18) -> (-77, -15) construction
  line L59 (-77, -15) -> (-73, -15) construction
  line L60 (-73, -15) -> (-73, -18) construction
  line L61 (-73, -18) -> (-71, -18) construction
  line L62 (-71, -18) -> (-71, -22) construction
  line L63 (-71, -22) -> (-73, -22) construction
  line L64 (-73, -22) -> (-73, -25) construction
  line L65 (-65, -25) -> (-73, -25) construction
  line L66 (-65, -25) -> (-65, -30) construction
  line L67 (-65, -30) -> (-45, -30) construction
  line L68 (-45, -30) -> (-45, -25) construction
  line L69 (-30, -25) -> (-45, -25) construction
  line L70 (-30, -30) -> (-30, -25) construction
  line L71 (30, -30) -> (-30, -30) construction
  line L72 (30, -25) -> (30, -30) construction
  line L73 (45, -25) -> (30, -25) construction
  line L74 (45, -30) -> (45, -25) construction
  line L75 (65, -30) -> (45, -30) construction
  line L76 (65, -25) -> (65, -30) construction
  line L77 (73, -25) -> (65, -25) construction
  line L78 (73, -25) -> (73, -22) construction
  line L79 (73, -22) -> (71, -22) construction
  line L80 (71, -22) -> (71, -18) construction
  line L81 (71, -18) -> (73, -18) construction
  line L82 (73, -18) -> (73, -15) construction
  line L83 (73, -15) -> (77, -15) construction
  line L84 (77, -15) -> (77, -18) construction
  line L85 (77, -18) -> (79, -18) construction
  line L86 (79, -18) -> (79, -22) construction
  line L87 (79, -22) -> (77, -22) construction
  line L88 (-45, -5) -> (-45, 15) construction
  line L89 (-45, 15) -> (-40, 15) construction
  line L90 (-40, 15) -> (-40, -5) construction
  line L91 (-40, -5) -> (-45, -5) construction
  circle A2 centre (42.5, 21) radius 2 construction
  circle A3 centre (-42.5, -11) radius 2 construction
  circle A4 centre (-42.5, 21) radius 2 construction
  circle A5 centre (42.5, -11) radius 2 construction
  line L92 (45, 15) -> (45, -5) construction
  line L93 (45, -5) -> (40, -5) construction
  line L94 (40, -5) -> (40, 15) construction
  line L95 (40, 15) -> (45, 15) construction
  circle A6 centre (0, 0) radius 11 construction
  circle A7 centre (75, 0) radius 4 construction
  circle A8 centre (-75, 0) radius 4 construction
  circle A9 centre (91, 0) radius 3 construction
  circle A10 centre (59, 0) radius 3 construction
  circle A11 centre (-59, 0) radius 3 construction
  circle A12 centre (-91, 0) radius 3 construction
  circle A13 centre (15.5, -15.5) radius 2.2846 construction
  circle A14 centre (-15.5, 15.5) radius 2 construction
  circle A15 centre (15.5, 15.5) radius 2 construction
  circle A16 centre (-15.5, -15.5) radius 2 construction
  line L96 (118, 15) -> (94, 15)
  line L97 (94, 15) -> (94, 22)
  line L98 (94, 22) -> (118, 22)
  line L99 (118, 22) -> (118, 15)
  point P0 (111, 17.5)
  dimension "d137" = 24
  dimension "d138" = 7
  dimension "d139" = 12
  dimension "d140" = 8
  constraints: 8 end point, 2 parallel, 1 horizontal, 1 perpendicular
  measures "d137" distance of L97.end L98.end
  measures "d138" distance of L96.end L97.end
  measures "d139" distance between parallel lines of L22 L99
  measures "d140" distance between parallel lines of L23 L98
extrude "Extrusion18" cut sketch "Sketch18" against normal blind 5
body "Solid3"
